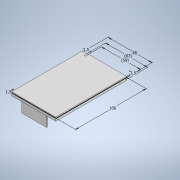
# Autodesk Inventor part: Bildschirm-Deckel.v3
Saved by Autodesk Inventor 2020 (Build 240168000, 168)
## iProperties
Created: 2019-08-24
Part Number: Bildschirm-Deckel.v3
Material: Generisch
Document SubType Name: Modeling
Designer: Admin
Density: 1 g/cm^3
Appearance: Vorgabe
Author: Admin
Autodesk Inventor part; units mm, degrees
ref_plane "YZ Plane" through (0, 0, 0) normal (1, 0, 0) x (0, 1, 0)
ref_plane "XZ Plane" through (0, 0, 0) normal (0, 1, 0) x (-1, 0, 0)
ref_plane "XY Plane" through (0, 0, 0) normal (0, 0, 1) x (1, 0, 0)
sketch "Skizze1" plane through (0, 0, 0) normal (0, 1, 0) x (-1, 0, 0)
  line L0 (0, 0) -> (66, 0)
  line L1 (66, 0) -> (66, 106)
  line L2 (66, 106) -> (0, 106)
  line L3 (0, 106) -> (0, 0)
  line L4 (66, 104.5) -> (0, 104.5)
  line L5 (64.5, 104.5) -> (64.5, 0)
  line L6 (1.5, 104.5) -> (1.5, 0)
  dimension "d0" = 106
  dimension "d1" = 66
  dimension "d2" = 1.5
  dimension "d3" = 1.5
  dimension "d4" = 1.5
  constraints: 14 end point, 6 point on line, 4 perpendicular, 2 parallel, 1 horizontal
  measures "d0" distance between parallel lines of L2 L0
  measures "d1" distance between parallel lines of L3 L1
  measures "d2" distance between parallel lines of L2 L4
  measures "d3" distance between parallel lines of L5 L1
  measures "d4" distance between parallel lines of L3 L6
extrude "Extrusion1" add sketch "Skizze1" along normal blind 1.5 contours L6 L4 L5 L0
extrude "Extrusion2" add sketch "Skizze1" along normal blind 1.5 and the other way blind 4 contours L3 L4 L6 L0 | L3 L2 L1 L4 | L5 L4 L1 L0
sketch "Skizze2" plane through (-1.5, -4, 0) normal (-1, 0, 0) x (0, 0, 1)
  line L0 (0, 0) -> (106, 0)
  line L1 (106, 0) -> (106, 1.5)
  line L2 (106, 1.5) -> (0, 1.5)
  line L3 (0, 1.5) -> (0, 0)
  point P0 (0, 4)
  dimension "d11" = 106
  dimension "d12" = 1.5
  constraints: 8 end point, 2 parallel, 1 horizontal, 1 perpendicular
  measures "d11" distance between parallel lines of L3 L1
  measures "d12" distance between parallel lines of L2 L0
extrude "Extrusion3" add sketch "Skizze2" along normal blind 2
sketch "Skizze3" plane through (-64.5, -4, 104.5) normal (1, 0, 0) x (0, 0, -1)
  point P0 (104.5, 4)
sketch "Skizze4" plane through (-64.5, -4, 104.5) normal (1, 0, 0) x (0, 0, -1)
  point P0 (104.5, 4)
sketch "Skizze5" plane through (-64.5, -4, 104.5) normal (1, 0, 0) x (0, 0, -1)
  line L0 (104.5676, 0) -> (-1.4324, 0)
  line L1 (-1.4324, 0) -> (-1.4324, 1.5)
  line L2 (-1.4324, 1.5) -> (104.5676, 1.5)
  line L3 (104.5676, 1.5) -> (104.5676, 0)
  point P0 (104.5, 4)
  dimension "d15" = 106
  dimension "d16" = 1.5
  dimension "d17" = 2.5
  constraints: 8 end point, 2 parallel, 1 horizontal, 1 perpendicular
  measures "d15" distance between parallel lines of L3 L1
  measures "d16" distance between parallel lines of L2 L0
  measures "d17" distance from line of L2 point (104.5, 4)
extrude "Extrusion4" add sketch "Skizze5" along normal blind 2
sketch "Skizze6" plane through (0, -4, 0) normal (0, -1, 0) x (1, 0, 0)
  line L0 (-3.5, 0) -> (-3.5, 104.5) projected
  line L1 (-62.5, 104.5) -> (-62.5, -0.0676) projected
  point P0 (0, 0)
  point P1 (-1.5, 0)
  point P2 (-64.5, 0)
  dimension "d20" = 59
  dimension "d21" = 63
  measures "d20" distance between parallel lines of L0 L1
  measures "d21" distance of point (-1.5, 0) point (-64.5, 0)
sketch "Skizze7" plane through (0, -4, 0) normal (0, -1, 0) x (1, 0, 0)
  line L0 (-51, 105.9518) -> (-14, 105.9518)
  line L1 (-14, 105.9518) -> (-14, 104.5031)
  line L2 (-14, 104.5031) -> (-51, 104.5031)
  line L3 (-51, 104.5031) -> (-51, 105.9518)
  line L4 (0, 0) -> (0, 106) projected
  line L5 (-66, 106) -> (-66, 0) projected
  dimension "d22" = 37
  dimension "d23" = 66
  dimension "d24" = 15
  constraints: 8 end point, 2 parallel, 1 horizontal, 1 perpendicular
  measures "d22" distance between parallel lines of L1 L3
  measures "d23" distance between parallel lines of L4 L5
  measures "d24" distance between parallel lines of L5 L3
extrude "Extrusion5" add sketch "Skizze7" along normal blind 15
